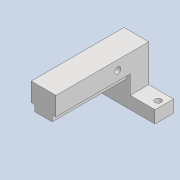
# Autodesk Inventor part: 0008-10-054 Suport doking
Saved by Autodesk Inventor 2020 (Build 240168000, 168)
## iProperties
Created: 2021-03-12
Part Number: 0008-10-054 Suport doking
Material: Generic
Document SubType Name: Modeling
Designer: Iulian Bors
Density: 1 g/cm^3
Appearance: Default
Description: Suport Doking
Mass: 29.9447 g
Surface Area: 87.7334 cm^2
Volume: 29.9447 cm^3
Author: Iulian Bors
Subject: 054
Autodesk Inventor part; units mm, degrees
ref_plane "YZ Plane" through (0, 0, 0) normal (1, 0, 0) x (0, 1, 0)
ref_plane "XZ Plane" through (0, 0, 0) normal (0, 1, 0) x (-1, 0, 0)
ref_plane "XY Plane" through (0, 0, 0) normal (0, 0, 1) x (1, 0, 0)
sketch "Sketch1" plane through (0, 0, 0) normal (0, 0, 1) x (1, 0, 0)
  line L0 (-30, 5) -> (30, 5)
  line L1 (30, 5) -> (30, -5)
  line L2 (30, -5) -> (-30, -5)
  line L3 (-30, -5) -> (-30, 5)
  line L4 (-10, 35) -> (10, 35)
  line L5 (10, 35) -> (10, 5)
  line L6 (10, 5) -> (-10, 5)
  line L7 (-10, 5) -> (-10, 35)
  point P0 (0, 0)
  point P1 (0, 5)
  point P2 (-30, 0)
  point P3 (0, 5)
  dimension "d0" = 10
  dimension "d1" = 60
  dimension "d2" = 30
  dimension "d3" = 20
  constraints: 16 end point, 4 parallel, 3 midpoint, 2 horizontal, 2 perpendicular, 1 coincident, 1 collinear, 1 horizontal alignment, 1 vertical alignment
  measures "d0" distance of L2.end L0.start
  measures "d1" distance of L0.start L0.end
  measures "d2" distance of L6.end L4.start
  measures "d3" distance of L4.start L4.end
extrude "Extrusion1" add sketch "Sketch1" along normal blind 15
sketch "Sketch2" plane through (-30, 5, 0) normal (0, 1, 0) x (1, 0, 0)
  line L0 (30, -53.7244) -> (30, -44.0936) construction
  line L1 (40, -15) -> (20, -15) construction
  line L2 (0, 0) -> (0, -15) projected
  point P0 (30, 0)
  point P1 (55, -7.5)
  point P2 (5, -7.5)
  point P3 (30, -48.909)
  point P4 (30, -15)
  point P5 (0, -7.5)
  dimension "d6" = 50
  constraints: 3 midpoint, 2 end point, 1 horizontal alignment, 1 symmetric about line, 1 vertical, 1 vertical alignment
  measures "d6" distance of point (5, -7.5) point (55, -7.5)
hole "Hole1" at (25, 5, 7.5) at (-25, 5, 7.5) direction (0, -1, 0) diameter 5 end through all
sketch "Sketch3" plane through (0, 0, 15) normal (0, 0, 1) x (1, 0, 0)
  line L0 (-10, 35) -> (10, 35)
  line L1 (10, 35) -> (10, 15)
  line L2 (10, 15) -> (-10, 15)
  line L3 (-10, 15) -> (-10, 35)
  line L4 (10, 35) -> (-10, 35) projected
  line L5 (10, 5) -> (10, 35) projected
  line L6 (-10, 35) -> (-10, 5) projected
  line L7 (-10, 20) -> (-7, 20)
  line L8 (-7, 20) -> (-7, 15)
  line L9 (-7, 15) -> (-10, 15)
  line L10 (-10, 15) -> (-10, 20)
  line L11 (7, 20) -> (10, 20)
  line L12 (10, 20) -> (10, 15)
  line L13 (10, 15) -> (7, 15)
  line L14 (7, 15) -> (7, 20)
  line L15 (10, 5) -> (10, 35) projected
  point P0 (0, 0)
  point P1 (-10, 20)
  dimension "d14" = 20
  dimension "d15" = 3
  dimension "d16" = 5
  constraints: 24 end point, 6 parallel, 5 collinear, 3 horizontal, 3 perpendicular, 2 equal length, 1 midpoint, 1 point on line
  measures "d14" distance of L2.end L0.start
  measures "d15" distance of L7.start L7.end
  measures "d16" distance of L7.end L8.end
extrude "Extrusion2" add sketch "Sketch3" along normal blind 35 contours L0 L1 L11 L14 L2 L8 L7 L3
sketch "Sketch4" plane through (-10, 5, 0) normal (-1, 0, 0) x (0, 0, 1)
  line L0 (50, 30) -> (50, 15) projected
  line L1 (15, 15) -> (15, 0) projected
  point P0 (0, -5)
  point P1 (25, 22.5)
  point P2 (50, 22.5)
  dimension "d27" = 25
  constraints: 1 horizontal alignment, 1 midpoint
  measures "d27" distance from line of L0 point (25, 22.5)
hole "Hole2" at (-10, 27.5, 25) direction (1, 0, 0) diameter 5 end through all counterbore diameter 9 counterbore depth 5
body "Solid1"
